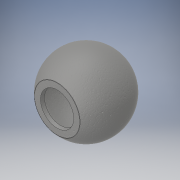
# Autodesk Inventor part: Lamp
Saved by Autodesk Inventor 2018.2 (Build 222227000, 227)
## iProperties
Created: 2018-01-26
Part Number: Lamp
Material: Beton
Document SubType Name: Modeling
Designer: JochenAlt
Density: 2.40731 g/cm^3
Appearance: Textur - grau
Author: JochenAlt
Autodesk Inventor part; units mm, degrees
ref_plane "YZ Plane" through (0, 0, 0) normal (1, 0, 0) x (0, 1, 0)
ref_plane "XZ Plane" through (0, 0, 0) normal (0, 1, 0) x (-1, 0, 0)
ref_plane "XY Plane" through (0, 0, 0) normal (0, 0, 1) x (1, 0, 0)
sketch "Skizze1" plane through (0, 0, 0) normal (0, 0, 1) x (1, 0, 0)
  line L0 (0, 95.3633) -> (0, -71.9553) construction
  line L1 (-14.8957, 0) -> (89.3745, 0) construction
  line L2 (6, 60.7042) -> (6, 49.6387)
  line L3 (26.5, -42.3999) -> (27.4875, -48)
  line L4 (37.2961, -48) -> (27.4875, -48)
  arc A0 (37.9177, -47.7833) -> (6, 60.7042) centre (0, 0) ccw
  arc A1 (26.5, -42.3999) -> (6, 49.6387) centre (0, 0) ccw
  arc A2 (37.2961, -48) -> (37.9177, -47.7833) centre (37.2961, -47) ccw
  point P0 (37.6431, -48)
  dimension "d3" = 6
  dimension "d7" = 26.5
  dimension "d8" = 1
  dimension "d10" = 50
  dimension "d11" = 61
  dimension "d12" = 10
  dimension "d13" = 48
  constraints: 7 point on circle, 6 end point, 3 centre point, 2 coincident, 2 tangent, 1 horizontal, 1 point on line, 1 vertical
  measures "d3" distance between parallel lines of L2 L0
  measures "d7" distance from line of L3.start L0
  measures "d8" radius of A2
  measures "d10" radius of A1
  measures "d11" radius of A0
  measures "d12" angle of L0 L3
  measures "d13" distance between parallel lines of L1 L4
revolve "Umdrehung1" add sketch "Skizze1" angle 360 about axis through (0, 0, 0) along (0, -1, 0)
